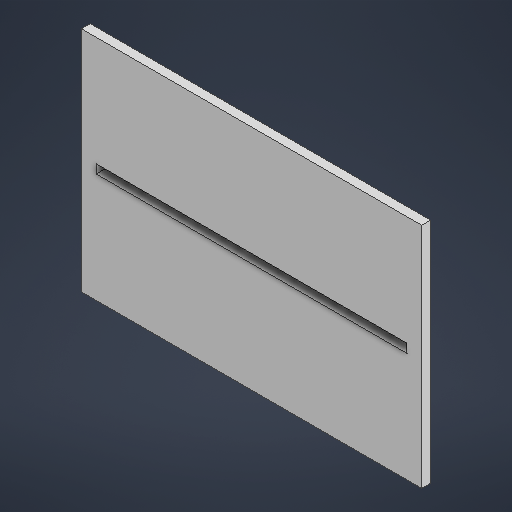
# Autodesk Inventor part: rampa
Saved by Autodesk Inventor 2026 (Build 300175000, 175)
## iProperties
Created: 2026-05-15
Part Number: rampa
Material: Generic
Document SubType Name: Modeling
Designer: juana
Density: 1 g/cm^3
Appearance: Default
Author: juana
Autodesk Inventor part; units mm, degrees
ref_plane "YZ Plane" through (0, 0, 0) normal (1, 0, 0) x (0, 1, 0)
ref_plane "XZ Plane" through (0, 0, 0) normal (0, 1, 0) x (-1, 0, 0)
ref_plane "XY Plane" through (0, 0, 0) normal (0, 0, 1) x (1, 0, 0)
sketch "Sketch1" plane through (0, 0, 0) normal (0, 0, 1) x (1, 0, 0)
  line L0 (0, 0) -> (0, 77)
  line L1 (0, 77) -> (115, 77)
  line L2 (115, 77) -> (115, 0)
  line L3 (115, 0) -> (0, 0)
  dimension "d0" = 77
  dimension "d1" = 115
  constraints: 8 end point, 3 perpendicular, 1 vertical
  measures "d0" distance of L1.end L2.end
  measures "d1" distance of L0.end L1.end
extrude "Extrusion1" add sketch "Sketch1" along normal blind 3
sketch "Sketch2" plane through (0, 0, 0) normal (0, 0, -1) x (-1, 0, 0)
  line L0 (-110, 40) -> (-5, 40)
  line L1 (-5, 40) -> (-5, 37)
  line L2 (-5, 37) -> (-110, 37)
  line L3 (-110, 37) -> (-110, 40)
  line L4 (0, 77) -> (0, 0) projected
  line L5 (-115, 0) -> (-115, 77) projected
  point P0 (-5, 38.5)
  point P1 (0, 38.5)
  dimension "d4" = 3
  dimension "d5" = 5
  dimension "d6" = 5
  constraints: 8 end point, 2 midpoint, 2 parallel, 1 horizontal, 1 horizontal alignment, 1 perpendicular
  measures "d4" distance of L0.end L1.end
  measures "d5" distance between parallel lines of L4 L1
  measures "d6" distance between parallel lines of L5 L3
extrude "Extrusion2" cut sketch "Sketch2" against normal blind 10
body "Solid1"
